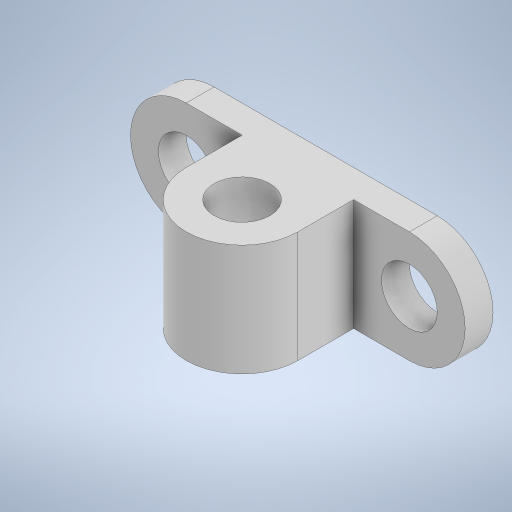
# Autodesk Inventor part: Part1
Saved by Autodesk Inventor 2024 (Build 280153000, 153)
## iProperties
Created: 2024-02-05
Part Number: Part1
Material: Generic
Document SubType Name: Modeling
Designer: rudyr
Density: 1 g/cm^3
Appearance: Default
Author: rudyr
Autodesk Inventor part; units mm, degrees
ref_plane "YZ Plane" through (0, 0, 0) normal (1, 0, 0) x (0, 1, 0)
ref_plane "XZ Plane" through (0, 0, 0) normal (0, 1, 0) x (-1, 0, 0)
ref_plane "XY Plane" through (0, 0, 0) normal (0, 0, 1) x (1, 0, 0)
sketch "Sketch1" plane through (0, 0, 0) normal (0, 0, 1) x (1, 0, 0)
  line L0 (0, 0) -> (80, 0)
  line L1 (0, 0) -> (50.337, 0)
  line L2 (0, 0) -> (80, 0)
  line L3 (80, 0) -> (80, 40)
  line L4 (80, 40) -> (0, 40)
  line L5 (0, 40) -> (0, 0)
  arc A0 (0, 40) -> (0, 0) centre (0, 20) ccw
  arc A1 (80, 0) -> (80, 40) centre (80, 20) ccw
  dimension "d1" = 80
  dimension "d2" = 40
  constraints: 12 end point, 4 point on circle, 2 centre point, 2 horizontal, 2 midpoint, 2 parallel, 1 perpendicular, 1 point on line
  measures "d1" distance of L4.end L3.end
  measures "d2" distance of L3.end L0.end
extrude "Extrusion1" add sketch "Sketch1" along normal blind 10
sketch "Sketch2" plane through (0, 0, 10) normal (0, 0, 1) x (1, 0, 0)
  arc A0 (0, 40) -> (0, 0) centre (0, 20) ccw projected
  circle A1 centre (0, 20) radius 10
  arc A2 (80, 0) -> (80, 40) centre (80, 20) ccw projected
  circle A3 centre (80, 20) radius 10
  dimension "d6" = 20
  dimension "d7" = 20
  constraints: 2 centre point, 2 coincident
  measures "d6" diameter of A1
  measures "d7" diameter of A3
extrude "Extrusion2" cut sketch "Sketch2" against normal blind 10
sketch "Sketch3" plane through (0, 0, 10) normal (0, 0, 1) x (1, 0, 0)
  line L0 (80, 40) -> (0, 40) projected
  line L1 (20, 40) -> (60, 40)
  line L2 (60, 40) -> (60, 0)
  line L3 (60, 0) -> (20, 0)
  line L4 (20, 0) -> (20, 40)
  arc A0 (0, 40) -> (0, 0) centre (0, 20) ccw projected
  dimension "d10" = 40
  dimension "d11" = 40
  dimension "d12" = 20
  constraints: 8 end point, 2 parallel, 1 horizontal, 1 perpendicular, 1 point on line
  measures "d10" distance of L2.end L3.end
  measures "d11" distance of L1.end L2.end
  measures "d12" horizontal distance of A0.centre L3.end
extrude "Extrusion3" add sketch "Sketch3" along normal blind 20
sketch "Sketch4" plane through (0, 0, 0) normal (0, -1, 0) x (1, 0, 0)
  line L0 (20, 30) -> (60, 30) projected
  arc A0 (60, 30) -> (20, 30) centre (40, 30) ccw
  point P0 (0, 0)
  constraints: 2 end point, 2 point on circle, 1 centre point, 1 midpoint
extrude "Extrusion4" add sketch "Sketch4" against normal blind 40
sketch "Sketch5" plane through (0, 0, 0) normal (0, -1, 0) x (1, 0, 0)
  arc A0 (60, 30) -> (20, 30) centre (40, 30) ccw projected
  circle A1 centre (40, 30) radius 10
  point P0 (0, 0)
  dimension "d17" = 20
  constraints: 1 centre point, 1 coincident
  measures "d17" diameter of A1
extrude "Extrusion5" cut sketch "Sketch5" against normal blind 40
body "Solid1"
